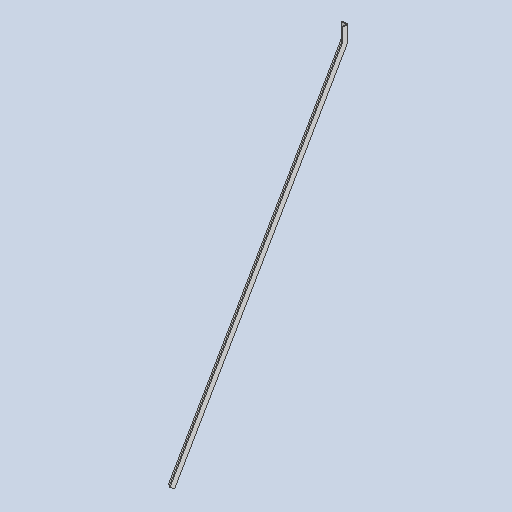
# Autodesk Inventor part: DiagL2
Saved by Autodesk Inventor 2023 (Build 270158030, 158C)
## iProperties
Created: 2022-07-29
Part Number: DiagL2
Material: Generic
Document SubType Name: Modeling
Designer: jeremyy
Density: 1 g/cm^3
Appearance: Default
Author: jeremyy
Autodesk Inventor part; units mm, degrees
ref_plane "YZ Plane" through (0, 0, 0) normal (1, 0, 0) x (0, 1, 0)
ref_plane "XZ Plane" through (0, 0, 0) normal (0, 1, 0) x (-1, 0, 0)
ref_plane "XY Plane" through (0, 0, 0) normal (0, 0, 1) x (1, 0, 0)
sketch "Sketch1" plane through (0, 0, 0) normal (1, 0, 0) x (0, 1, 0)
  line L0 (0, 0) -> (989.867, -571.5)
  line L1 (989.867, -571.5) -> (980.342, -587.9978)
  line L2 (980.342, -587.9978) -> (-9.525, -16.4978)
  line L3 (-9.525, -16.4978) -> (0, 0)
  line L4 (0, 0) -> (51.1145, 0)
  line L5 (980.342, -587.9978) -> (1031.142, -587.9978)
  line L6 (1031.142, -587.9978) -> (1031.142, -568.9478)
  line L7 (989.867, -571.5) -> (991.3406, -568.9478)
  line L8 (1031.142, -568.9478) -> (991.3406, -568.9478)
  line L9 (-9.525, -16.4978) -> (-7.9375, -13.7482)
  line L10 (-7.9375, -13.7482) -> (981.9295, -585.2482)
  line L11 (1031.142, -587.9978) -> (1031.142, -584.8228)
  line L12 (1031.142, -584.8228) -> (982.1751, -584.8228)
  dimension "d0" = 1143
  dimension "d1" = 19.05
  dimension "d2" = 1143
  dimension "d3" = 30
  dimension "d4" = 50.8
  dimension "d5" = 19.05
  dimension "d6" = 3.175
  dimension "d7" = 1143
  dimension "d8" = 3.175
  constraints: 26 end point, 5 point on line, 4 perpendicular, 3 horizontal
  measures "d0" distance of L0.start L0.end
  measures "d1" distance of L0.end L1.end
  measures "d2" distance of L1.end L2.end
  measures "d3" angle of L4 L0
  measures "d4" distance of L1.end L5.end
  measures "d5" distance of L5.end L6.end
  measures "d6" distance of L2.end L9.end
  measures "d7" distance of L9.end L10.end
  measures "d8" distance of L5.end L11.end
extrude "Extrusion1" add sketch "Sketch1" along normal blind 3.175
extrude "Extrusion2" add sketch "Sketch1" against normal blind 15.875 contours L10 L1 L2 L3 | L12 L6 L5 L1
body "Solid1"
